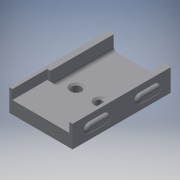
# Autodesk Inventor part: Top
Saved by Autodesk Inventor 2018 (Build 220112000, 112)
## iProperties
Created: 2018-05-15
Part Number: Top
Material: Generic
Document SubType Name: Modeling
Designer: Mandus
Density: 1 g/cm^3
Appearance: Default
Author: Mandus
Autodesk Inventor part; units mm, degrees
ref_plane "YZ Plane" through (0, 0, 0) normal (1, 0, 0) x (0, 1, 0)
ref_plane "XZ Plane" through (0, 0, 0) normal (0, 1, 0) x (-1, 0, 0)
sketch "Sketch1" plane through (0, 0, 0) normal (0, 0, 1) x (1, 0, 0)
  line L0 (0, 0) -> (20, 0)
  line L1 (20, 0) -> (20, 31)
  line L2 (20, 31) -> (0, 31)
  line L3 (0, 31) -> (0, 0)
  dimension "d0" = 20
  dimension "d1" = 31
  constraints: 8 end point, 2 parallel, 1 horizontal, 1 perpendicular
  measures "d0" distance of L2.end L1.end
  measures "d1" distance of L1.end L0.end
extrude "Extrusion1" add sketch "Sketch1" along normal blind 7
sketch "Sketch2" plane through (0, 0, 7) normal (0, 0, 1) x (1, 0, 0)
  line L0 (20, 31) -> (0, 31) projected
  line L1 (2, 31) -> (18, 31)
  line L2 (18, 31) -> (18, 11)
  line L3 (18, 11) -> (2, 11)
  line L4 (2, 11) -> (2, 31)
  line L5 (0, 31) -> (0, 0) projected
  line L6 (20, 0) -> (20, 31) projected
  dimension "d4" = 20
  dimension "d5" = 2
  dimension "d6" = 2
  constraints: 8 end point, 2 parallel, 1 horizontal, 1 perpendicular, 1 point on line
  measures "d4" distance of L1.end L2.end
  measures "d5" distance from line of L5 L1.start
  measures "d6" distance from line of L6 L1.end
extrude "Extrusion2" cut sketch "Sketch2" against normal blind 4.5
sketch "Sketch3" plane through (0, 0, 7) normal (0, 0, 1) x (1, 0, 0)
  line L0 (18, 11) -> (2, 11) projected
  line L1 (1, 0) -> (19, 0)
  line L2 (19, 0) -> (19, 11)
  line L3 (19, 11) -> (1, 11)
  line L4 (1, 11) -> (1, 0)
  line L5 (0, 31) -> (0, 0) projected
  line L6 (20, 0) -> (20, 31) projected
  dimension "d9" = 1
  dimension "d10" = 1
  constraints: 8 end point, 2 parallel, 1 horizontal, 1 perpendicular, 1 point on line
  measures "d9" distance from line of L5 L1.start
  measures "d10" distance from line of L6 L1.end
extrude "Extrusion3" cut sketch "Sketch3" against normal blind 3
sketch "Sketch4" plane through (0, 0, 2.5) normal (0, 0, 1) x (1, 0, 0)
  circle A0 centre (6.19, 15) radius 1.5
  circle A1 centre (13.81, 15) radius 1.5
  line L0 (19, 0) -> (1, 0) projected
  line L1 (2, 31) -> (18, 31) projected
  line L2 (2, 11) -> (2, 31) construction
  line L3 (2, 31) -> (18, 31) construction
  line L4 (2, 11) -> (2, 31) construction
  line L5 (18, 11) -> (2, 11) construction
  line L6 (18, 31) -> (18, 11) construction
  line L7 (20, 31) -> (0, 31) construction
  line L8 (10, 31) -> (10, 11) construction
  line L9 (18, 11) -> (2, 11) construction
  line L10 (10, 31) -> (30, 31) construction
  point P0 (0, 0)
  point P1 (2, 21)
  dimension "d13" = 3
  dimension "d14" = 3
  dimension "d15" = 7.62
  dimension "d16" = 15
  dimension "d17" = 90
  constraints: 4 end point, 3 midpoint, 2 centre point, 1 horizontal, 1 horizontal alignment, 1 perpendicular, 1 symmetric about line
  measures "d13" diameter of A0
  measures "d14" diameter of A1
  measures "d15" distance of A1.centre A0.centre
  measures "d16" distance from line of L0 A0.centre
  measures "d17" angle of L8 L10
extrude "Extrusion4" cut sketch "Sketch4" against normal up to next
chamfer "Chamfer1" distance 0.5 angle 45 2 edges at (4.69, 15, 2.5) (12.31, 15, 2.5)
sketch "Sketch5" plane through (20, 0, 0) normal (1, 0, 0) x (0, 0, -1)
  line L0 (0, 0) -> (-7, 0) construction
  line L1 (-3.5, 0) -> (-3.5, 31) construction
  line L2 (-3.5, 0) -> (27.5, 0) construction
  line L3 (-3.5, 5) -> (-3.5, 10) construction
  line L4 (-2, 5) -> (-2, 10)
  line L5 (-5, 10) -> (-5, 5)
  arc A0 (-5, 5) -> (-2, 5) centre (-3.5, 5) ccw
  arc A1 (-2, 10) -> (-5, 10) centre (-3.5, 10) ccw
  line L6 (-3.5, 21) -> (-3.5, 26) construction
  line L7 (-2, 21) -> (-2, 26)
  line L8 (-5, 26) -> (-5, 21)
  arc A2 (-5, 21) -> (-2, 21) centre (-3.5, 21) ccw
  arc A3 (-2, 26) -> (-5, 26) centre (-3.5, 26) ccw
  line L9 (0, 31) -> (-7, 31) projected
  point P0 (-3.5, 7.5)
  point P1 (-3.5, 23.5)
  dimension "d23" = 31
  dimension "d24" = 90
  dimension "d25" = 3
  dimension "d26" = 3
  dimension "d27" = 5
  dimension "d28" = 5
  dimension "d29" = 5
  dimension "d30" = 5
  constraints: 20 end point, 8 point on circle, 8 tangent, 4 centre point, 4 point on line, 3 midpoint, 2 parallel, 1 horizontal, 1 perpendicular, 1 vertical
  measures "d23" distance of L1.start L1.end
  measures "d24" angle of L2 L1
  measures "d25" diameter of A1
  measures "d26" diameter of A3
  measures "d27" distance from line of L9 L6.end
  measures "d28" distance of L6.start L6.end
  measures "d29" distance from line of L2 L3.start
  measures "d30" distance of L3.start L3.end
extrude "Extrusion5" add sketch "Sketch5" along normal blind 1
ref_plane "Work Plane1" through (10, 0, 0) normal (1, 0, 0) x (0, 0, -1)
mirror "Mirror1" about plane through (10, 0, 0) normal (1, 0, 0) of "Extrusion5"
fillet "Fillet2" radius 1 16 edges at (21, 19.5, 3.5) (21, 23.5, 2) (21, 27.5, 3.5) (21, 23.5, 5) (21, 3.5, 3.5) (21, 7.5, 2) (21, 11.5, 3.5) (21, 7.5, 5) (-1, 19.5, 3.5) (-1, 23.5, 2) (-1, 27.5, 3.5) (-1, 23.5, 5) (-1, 3.5, 3.5) (-1, 7.5, 2) (-1, 11.5, 3.5) (-1, 7.5, 5)
fillet "Fillet3" radius 1 2 edges at (2, 21, 2.5) (18, 21, 2.5)
chamfer "Chamfer2" distance 0.5 angle 45 2 edges at (12.31, 15, 0) (4.69, 15, 0)
body "Solid1"
